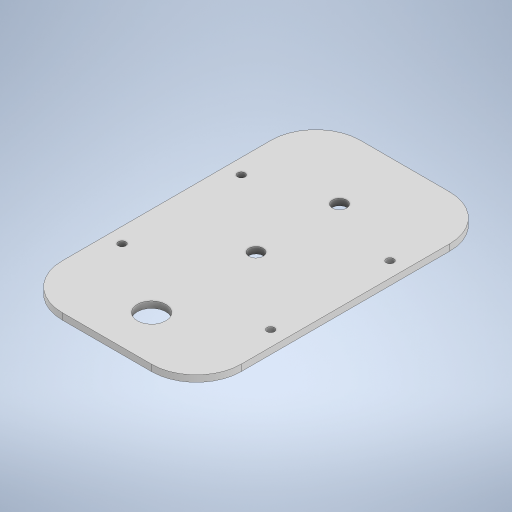
# Autodesk Inventor part: Plate
Saved by Autodesk Inventor 2024 (Build 280153000, 153)
## iProperties
Created: 2024-01-20
Part Number: Plate
Material: Generic
Document SubType Name: Modeling
Designer: Irwin
Density: 1 g/cm^3
Appearance: Default
Author: Irwin
Autodesk Inventor part; units mm, degrees
ref_plane "YZ Plane" through (0, 0, 0) normal (1, 0, 0) x (0, 1, 0)
ref_plane "XZ Plane" through (0, 0, 0) normal (0, 1, 0) x (-1, 0, 0)
ref_plane "XY Plane" through (0, 0, 0) normal (0, 0, 1) x (1, 0, 0)
sketch "Sketch1" plane through (0, 0, 0) normal (0, 1, 0) x (-1, 0, 0)
  line L0 (-75, 125) -> (75, 125)
  line L1 (75, 125) -> (75, -125)
  line L2 (75, -125) -> (-75, -125)
  line L3 (-75, -125) -> (-75, 125)
  line L4 (-75, 125) -> (75, -125) construction
  line L5 (75, 125) -> (-75, -125) construction
  point P0 (0, 0)
  dimension "d0" = 150
  dimension "d1" = 250
  constraints: 12 end point, 2 midpoint, 2 parallel, 1 horizontal, 1 perpendicular
  measures "d0" distance of L1.end L2.end
  measures "d1" distance of L0.end L1.end
extrude "Extrusion1" add sketch "Sketch1" along normal blind 5.4
fillet "Fillet1" radius 37.5 4 edges at (75, 2.7, 125) (75, 2.7, -125) (-75, 2.7, 125) (-75, 2.7, -125)
sketch "Sketch2" plane through (0, 5.4, 0) normal (0, 1, 0) x (1, 0, 0)
  line L0 (37.5, -125) -> (-37.5, -125)
  line L1 (-37.5, -125) -> (-37.5, -50)
  line L2 (-37.5, -50) -> (37.5, -50)
  line L3 (37.5, -50) -> (37.5, -125)
  line L4 (-37.5, -125) -> (37.5, -125) projected
  line L5 (-75, 87.5) -> (-75, -87.5) projected
  circle A0 centre (0, -87.5) radius 12
  point P0 (0, 0)
  point P1 (-37.5, -87.5)
  point P2 (0, -50)
  dimension "d6" = 75
  dimension "d7" = 0
  dimension "d9" = 24
  dimension "d10" = 37.5
  dimension "d11" = 37.5
  constraints: 8 end point, 2 midpoint, 2 parallel, 2 vertical alignment, 1 centre point, 1 horizontal, 1 perpendicular
  measures "d6" distance of L0.end L1.end
  measures "d7" distance between parallel lines of L4 L0
  measures "d9" diameter of A0
  measures "d10" distance of point (-37.5, -87.5) A0.centre
  measures "d11" distance of point (0, -50) A0.centre
extrude "Extrusion2" cut sketch "Sketch2" against normal blind 20.5 contours A0
sketch "Sketch3" plane through (0, 5.4, 0) normal (0, 1, 0) x (1, 0, 0)
  circle A0 centre (0, 0) radius 6
  circle A1 centre (0, 70) radius 6
  line L0 (37.5, 125) -> (-37.5, 125) projected
  line L1 (-75, 87.5) -> (-75, -87.5) projected
  line L2 (-37.5, -125) -> (37.5, -125) projected
  line L3 (75, -87.5) -> (75, 87.5) projected
  point P0 (0, 125)
  point P1 (0, 125)
  point P2 (0, -125)
  dimension "d15" = 12
  dimension "d16" = 55
  dimension "d21" = 75
  dimension "d22" = 125
  dimension "d23" = 250
  dimension "d24" = 150
  constraints: 3 midpoint, 2 centre point, 1 equal radius, 1 vertical alignment
  measures "d15" diameter of A1
  measures "d16" distance from line of L0 A1.centre
  measures "d21" distance from line of L1 A0.centre
  measures "d22" distance of point (0, 125) A0.centre
  measures "d23" distance of point (0, 125) point (0, -125)
  measures "d24" distance between parallel lines of L3 L1
extrude "Extrusion3" cut sketch "Sketch3" against normal blind 40
sketch "Sketch4" plane through (0, 5.4, 0) normal (0, 1, 0) x (1, 0, 0)
  circle A0 centre (-62.3, 50) radius 3.175
  line L0 (37.5, 125) -> (-37.5, 125) projected
  line L1 (-75, 87.5) -> (-75, -87.5) projected
  circle A1 centre (-62.3, -50) radius 3.175
  circle A2 centre (62.3, 50) radius 3.175
  circle A3 centre (62.3, -50) radius 3.175
  point P0 (0, 0)
  dimension "d27" = 100
  dimension "d30" = 124.6
  dimension "d33" = 12.7
  dimension "d34" = 6.35
  dimension "d35" = 50
  constraints: 4 centre point, 1 horizontal, 1 vertical, 6 other
  measures "d27" distance of A0.centre A1.centre
  measures "d30" distance of A0.centre A2.centre
  measures "d33" distance from line of L1 A0.centre
  measures "d34" diameter of A0
  measures "d35" vertical distance of point (0, 0) A0.centre
extrude "Extrusion4" cut sketch "Sketch4" against normal blind 40
equation "\"d21\" = 0.5 * d24"
equation "\"d22\" = 0.5 * d23"
equation "\"d27\" = 2 * d35"
body "Solid1"
